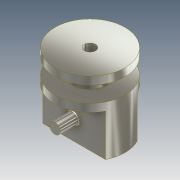
# Autodesk Inventor part: slider-1
Saved by Autodesk Inventor 2017 (Build 210142000, 142)
## iProperties
Created: 2018-05-30
Part Number: slider-1
Material: Generic
Document SubType Name: Modeling
Designer: Luiz Gustavo
Density: 1 g/cm^3
Appearance: Silver
Mass: 3.87628 g
Surface Area: 25.457 cm^2
Volume: 3.87628 cm^3
Author: Luiz Gustavo
Autodesk Inventor part; units mm, degrees
ref_plane "YZ Plane" through (0, 0, 0) normal (1, 0, 0) x (0, 1, 0)
ref_plane "XZ Plane" through (0, 0, 0) normal (0, 1, 0) x (-1, 0, 0)
ref_plane "XY Plane" through (0, 0, 0) normal (0, 0, 1) x (1, 0, 0)
sketch "Sketch1" plane through (0, 0, 0) normal (0, 0, 1) x (1, 0, 0)
  arc A0 (-8.9303, 4.5) -> (-8.9303, -4.5) centre (0, 0) ccw
  circle A1 centre (0, 0) radius 4.5 construction
  line L0 (-8.9303, 4.5) -> (8.9303, 4.5)
  line L1 (-8.9303, -4.5) -> (8.9303, -4.5)
  arc A2 (8.9303, 4.5) -> (-8.9303, 4.5) centre (0, 0) ccw
  arc A3 (8.9303, -4.5) -> (8.9303, 4.5) centre (0, 0) ccw
  arc A4 (-8.9303, -4.5) -> (8.9303, -4.5) centre (0, 0) ccw
  dimension "d0" = 20
  dimension "d1" = 9
  constraints: 9 point on circle, 5 centre point, 4 end point, 2 coincident, 2 horizontal, 2 tangent
  measures "d0" diameter of A0
  measures "d1" diameter of A1
extrude "Extrusion1" add sketch "Sketch1" against normal blind 12 contours L0 A3 L1 A0
extrude "Extrusion2" add sketch "Sketch1" along normal blind 9
sketch "Sketch2" plane through (0, 0, 0) normal (0, 1, 0) x (-1, 0, 0)
  circle A0 centre (0, -6) radius 1.5
  line L0 (0, 0) -> (0, -6) construction
  dimension "d6" = 3
  dimension "d7" = 6
  constraints: 2 end point, 1 centre point, 1 vertical
  measures "d6" diameter of A0
  measures "d7" distance of L0.end L0.start
extrude "Extrusion3" add sketch "Sketch2" along normal mid plane 20
sketch "Sketch3" plane through (0, 0, 0) normal (0, 1, 0) x (-1, 0, 0)
  line L0 (10, 9) -> (-10, 9) construction
  line L1 (8.9303, 0) -> (-8.9303, 0) construction
  line L2 (0, 9) -> (0, 0) construction
  line L3 (-8.9303, 0) -> (8.9303, 0) construction
  line L4 (0, 4.5) -> (-10, 4.5) construction
  line L5 (-10, 9) -> (-10, -12) construction
  line L6 (-5, 2.25) -> (-10, 2.25)
  line L7 (-10, 2.25) -> (-10, 6.75)
  line L8 (-10, 6.75) -> (-5, 6.75)
  line L9 (-5, 6.75) -> (-5, 2.25)
  line L10 (-5, 2.25) -> (-10, 6.75) construction
  line L11 (-10, 2.25) -> (-5, 6.75) construction
  point P0 (-7.5, 4.5)
  dimension "d10" = 4.5
  dimension "d11" = 10
  constraints: 16 end point, 4 midpoint, 2 horizontal, 2 parallel, 2 perpendicular, 2 point on line, 1 collinear
  measures "d10" distance of L8.end L6.start
  measures "d11" diameter of L9 L2
revolve "Revolution1" cut sketch "Sketch3" angle 360 about axis through (0, 0, 9) along (0, 0, -1)
sketch "Sketch4" plane through (0, 0, 0) normal (0, 0, 1) x (1, 0, 0)
  circle A0 centre (0, 0) radius 1.6
  dimension "d22" = 3.2
  constraints: 1 centre point, 1 coincident
  measures "d22" diameter of A0
extrude "Extrusion4" cut sketch "Sketch4" along normal through all both and the other way through all
chamfer "Chamfer1" [suppressed]
fillet "Fillet1" radius 0.5 2 edges at (1.5, -4.5, -6) (1.5, 4.5, -6)
body "Solid1"
